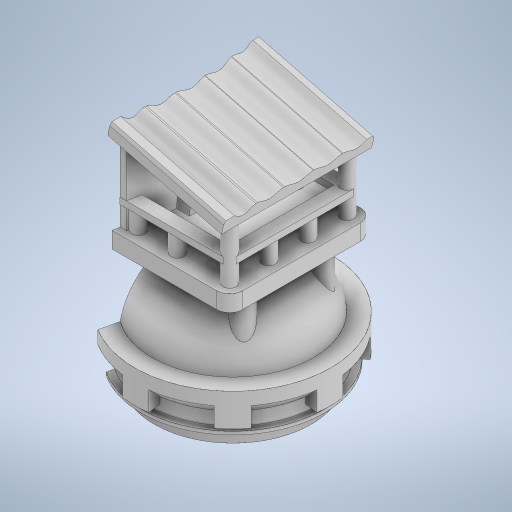
# Autodesk Inventor part: 不知道取啥
Saved by Autodesk Inventor 2024 (Build 280153000, 153)
## iProperties
Created: 2024-05-19
Part Number: 不知道取啥
Material: 一般
Document SubType Name: Modeling
Designer: User
Density: 1 g/cm^3
Appearance: 預設
Author: User
Autodesk Inventor part; units mm, degrees
ref_plane "YZ Plane" through (0, 0, 0) normal (1, 0, 0) x (0, 1, 0)
ref_plane "XZ Plane" through (0, 0, 0) normal (0, 1, 0) x (-1, 0, 0)
ref_plane "XY Plane" through (0, 0, 0) normal (0, 0, 1) x (1, 0, 0)
sketch "草圖1" plane through (0, 0, 0) normal (0, 1, 0) x (-1, 0, 0)
  circle A0 centre (0, 0) radius 15
  dimension "d0" = 30
  constraints: 1 centre point, 1 coincident
  measures "d0" diameter of A0
extrude "擠出1" add sketch "草圖1" along normal blind 2
sketch "草圖2" plane through (0, 0, 0) normal (0, 0, 1) x (1, 0, 0)
  line L0 (0, 0) -> (0, -2)
  line L1 (15, 0) -> (-15, 0) projected
  line L2 (0, -2) -> (13, -2)
  line L3 (13, -2) -> (15, 0)
  dimension "d3" = 2
  dimension "d5" = 13
  constraints: 6 end point, 1 horizontal, 1 vertical
  measures "d3" distance of L0.start L0.end
  measures "d5" distance of L0.end L2.end
sketch "草圖3" plane through (0, 0, 0) normal (0, -1, 0) x (1, 0, 0)
  circle A0 centre (0, 0) radius 15
  circle A1 centre (0, 0) radius 13
  line L0 (0, 0) -> (2, 14.866069)
  line L1 (0, 0) -> (-2, 14.866069)
  line L2 (-2, 14.866069) -> (2, 14.866069)
  line L3 (0, 0) -> (-9.097684, 11.926112)
  line L4 (0, 0) -> (-11.926112, 9.097684)
  line L5 (0, 0) -> (-14.866069, 2)
  line L6 (0, 0) -> (-14.866069, -2)
  line L7 (0, 0) -> (-11.926112, -9.097684)
  line L8 (0, 0) -> (-9.097684, -11.926112)
  line L9 (0, 0) -> (-2, -14.866069)
  line L10 (0, 0) -> (2, -14.866069)
  line L11 (0, 0) -> (9.097684, -11.926112)
  line L12 (0, 0) -> (11.926112, -9.097684)
  line L13 (0, 0) -> (14.866069, -2)
  line L14 (0, 0) -> (14.866069, 2)
  line L15 (0, 0) -> (11.926112, 9.097684)
  line L16 (0, 0) -> (9.097684, 11.926112)
  point P0 (1.733333, -12.883926)
  point P1 (-1.733333, -12.883926)
  point P2 (-7.88466, -10.335963)
  point P3 (-10.335963, -7.88466)
  point P4 (-12.883926, -1.733333)
  point P5 (-12.883926, 1.733333)
  point P6 (10.335963, -7.88466)
  point P7 (7.88466, -10.335963)
  point P8 (12.883926, 1.733333)
  point P9 (12.883926, -1.733333)
  point P10 (7.88466, 10.335963)
  point P11 (10.335963, 7.88466)
  point P12 (-10.335963, 7.88466)
  point P13 (-7.88466, 10.335963)
  point P14 (-1.733333, 12.883926)
  point P15 (1.733333, 12.883926)
  dimension "d4" = 30
  dimension "d6" = 26
  dimension "d7" = 4
  dimension "d8" = 82.3377
  dimension "d9" = 82.3377
  dimension "d12" = 360
  constraints: 34 end point, 4 coincident, 2 centre point, 2 point on circle, 1 horizontal, 39 other
  measures "d4" diameter of A0
  measures "d6" diameter of A1
  measures "d7" distance of L0.end L1.end
  measures "d8" angle of L0 L2
  measures "d9" angle of L1 L2
extrude "擠出2" add sketch "草圖3" along normal blind 3 contours A0 L13 A1 L14 | L15 A1 L16 A0 | A0 L11 A1 L12 | L2 A0 | L0 A1 L1 L2 | A1 L4 A0 L3 | A1 L6 A0 L5 | A1 L8 A0 L7 | A1 L10 A0 L9
revolve "迴轉1" add sketch "草圖2" angle 360 about axis through (0, 0, 0) along (0, -1, 0)
sketch "草圖4" plane through (0, -2, 0) normal (0, -1, 0) x (1, 0, 0)
  circle A0 centre (0, 0) radius 13
  dimension "d17" = 26
  constraints: 1 centre point, 1 coincident
  measures "d17" diameter of A0
extrude "擠出3" add sketch "草圖4" along normal blind 2
sketch "草圖5" plane through (0, -4, 0) normal (0, -1, 0) x (1, 0, 0)
  circle A0 centre (0, 0) radius 14
  dimension "d20" = 28
  constraints: 1 centre point, 1 coincident
  measures "d20" diameter of A0
extrude "擠出4" add sketch "草圖5" along normal blind 0.5
sketch "草圖6" plane through (0, 0, 0) normal (1, 0, 0) x (0, 1, 0)
  line L0 (-4.5, 14) -> (-4.5, -14) projected
  line L1 (-4.5, 0) -> (-4.5, -13)
  line L2 (-4.5, -13) -> (-7, -12)
  line L3 (-7, -12) -> (-7, 0)
  line L4 (-7, 0) -> (-4.5, 0)
  point P0 (0, 0)
  dimension "d23" = 13
  dimension "d24" = 12
  dimension "d25" = 2.5
  constraints: 8 end point, 1 midpoint, 1 parallel, 1 perpendicular, 1 point on line
  measures "d23" distance of L1.start L1.end
  measures "d24" distance of L2.end L3.end
  measures "d25" distance between parallel lines of L0 L3
revolve "迴轉2" add sketch "草圖6" angle 360 about axis through (0, -7, 0) along (0, 1, 0)
ref_plane "工作平面1" through (0, 0, 0) normal (0, 1, 0) x (1, 0, 0)
sketch "草圖7" plane through (0, 0, 0) normal (0, 1, 0) x (1, 0, 0)
  circle A0 centre (0, 0) radius 12.5
  line L0 (-12.5, 0) -> (13, 0)
  arc A1 (12.883926, -1.733333) -> (12.883926, 1.733333) centre (0, 0) ccw
  point P0 (12.5, 0)
  dimension "d28" = 25
  constraints: 2 end point, 1 coincident, 1 horizontal, 1 point on circle, 3 other
revolve "迴轉3" add sketch "草圖7" angle 180 about axis through (-12.5, 0, 0) along (1, 0, 0) picked at (-2.404316, 7.656061) contours L0 A0
sketch "草圖8" plane through (0, 2, 0) normal (0, 1, 0) x (1, 0, 0)
  circle A0 centre (7.515021, -6) radius 1.5
  circle A1 centre (7.515021, 6) radius 1.5
  line L0 (0, 0) -> (8.693271, 0)
  dimension "d30" = 3
  dimension "d31" = 3
  dimension "d32" = 6
  dimension "d33" = 6
  constraints: 2 centre point, 2 end point, 1 horizontal
  measures "d30" diameter of A0
  measures "d31" diameter of A1
  measures "d32" distance from line of L0 A0.centre
  measures "d33" distance from line of L0 A1.centre
extrude "擠出5" add sketch "草圖8" along normal blind 10
sketch "草圖9" plane through (7.515021, 12, 6) normal (0, 1, 0) x (1, 0, 0)
  line L0 (1, -5) -> (-15, -5)
  line L1 (-15, -5) -> (-15, 17)
  line L2 (-15, 17) -> (1, 17)
  line L3 (3, 15) -> (3, -3)
  arc A0 (1, -5) -> (3, -3) centre (1, -3) ccw
  arc A1 (3, 15) -> (1, 17) centre (1, 15) ccw
  circle A2 centre (0, 0) radius 1.5
  circle A3 centre (0, 12) radius 1.5
  line L4 (0, 0) -> (0, 12)
  line L5 (0, 6) -> (-5.052859, 6)
  point P0 (-7.515021, 6)
  point P1 (3, -5)
  dimension "d36" = 22
  dimension "d37" = 18
  dimension "d38" = 2
  dimension "d39" = 11
  dimension "d40" = 3
  constraints: 12 end point, 4 point on circle, 4 tangent, 2 centre point, 2 horizontal, 2 parallel, 2 point on line, 1 equal radius, 1 midpoint, 1 perpendicular, 1 vertical
  measures "d36" distance of L0.end L1.end
  measures "d37" distance of point (3, -5) L0.end
  measures "d38" radius of A0
  measures "d39" distance between parallel lines of L2 L5
  measures "d40" distance between parallel lines of L4 L3
extrude "擠出6" add sketch "草圖9" along normal blind 2.5 contours L0 L1 L2 A1 L3 A0 | A2 | A3
sketch "草圖10" plane through (7.515021, 14.5, 6) normal (0, 1, 0) x (1, 0, 0)
  circle A0 centre (1, -3) radius 1
  circle A1 centre (1, 15) radius 1
  arc A2 (1, -5) -> (3, -3) centre (1, -3) ccw projected
  arc A3 (3, 15) -> (1, 17) centre (1, 15) ccw projected
  circle A4 centre (-7, -3) radius 1
  circle A5 centre (-13, -3) radius 1
  circle A6 centre (1, 3) radius 1
  circle A7 centre (1, 9) radius 1
  circle A8 centre (-7, 15) radius 1
  circle A9 centre (-13, 15) radius 1
  point P0 (-7.515021, 6)
  dimension "d43" = 2
  dimension "d44" = 2
  dimension "d45" = 2
  dimension "d46" = 2
  dimension "d47" = 2
  dimension "d48" = 2
  dimension "d49" = 6
  dimension "d50" = 6
  dimension "d51" = 8
  dimension "d52" = 6
  dimension "d53" = 2
  dimension "d54" = 2
  constraints: 8 centre point, 2 concentric
  measures "d43" diameter of A0
  measures "d44" diameter of A1
  measures "d45" diameter of A4
  measures "d46" diameter of A5
  measures "d47" diameter of A6
  measures "d48" diameter of A7
  measures "d49" distance of A0.centre A6.centre
  measures "d50" distance of A1.centre A7.centre
  measures "d51" distance of A4.centre A0.centre
  measures "d52" distance of A5.centre A4.centre
  measures "d53" diameter of A8
  measures "d54" diameter of A9
extrude "擠出7" add sketch "草圖10" along normal blind 3
sketch "草圖11" plane through (8.515021, 17.5, -9) normal (0, 1, 0) x (1, 0, 0)
  circle A0 centre (0, -18) radius 1
  line L0 (1, -18) -> (1, 0)
  circle A1 centre (0, 0) radius 1
  line L1 (0, 1) -> (-15.99965, 1)
  line L2 (0, 2) -> (-16, 2)
  line L3 (-15.99965, 1) -> (-15.99965, -1)
  line L4 (-1, -12.008919) -> (-1, -1)
  line L5 (-1, -1) -> (-15.99965, -1)
  line L6 (0, -19) -> (-16, -19)
  line L7 (-16, -19) -> (-16, -17)
  line L8 (-16, -17) -> (-1, -17)
  line L9 (-1, -17) -> (-1, -12.008919)
  circle A2 centre (0, 0) radius 1
  circle A3 centre (0, -18) radius 1
  point P0 (-8.515021, -9)
  point P1 (0, 1)
  dimension "d57" = 2
  dimension "d58" = 2
  constraints: 18 end point, 4 perpendicular, 3 point on circle, 3 tangent, 2 parallel, 2 vertical, 1 collinear, 1 point on line, 2 other
  measures "d57" distance of L1.end L3.end
  measures "d58" distance of L6.end L7.end
extrude "擠出8" add sketch "草圖11" along normal blind 1
sketch "草圖12" plane through (8.515021, 18.5, -9) normal (0, 1, 0) x (1, 0, 0)
  circle A0 centre (0, 0) radius 1
  arc A1 (1, -18) -> (0, -19) centre (0, -18) ccw projected
  circle A2 centre (0, -18) radius 1
  point P0 (-8.515021, -9)
  constraints: 2 centre point, 1 coincident
extrude "擠出9" add sketch "草圖12" along normal blind 4.9
ref_plane "工作平面2" through (8.515021, 17.5, 0) normal (0, 0, -1) x (-1, 0, 0)
sketch "草圖13" plane through (8.515021, 17.5, 0) normal (0, 0, -1) x (-1, 0, 0)
  line L0 (-1.734486, 7.276923) -> (-1.240987, 5.338764)
  line L1 (-1.240987, 5.338764) -> (16.202441, 9.78025)
  line L2 (-1.734486, 7.276923) -> (15.708943, 11.718409)
  line L3 (15.708943, 11.718409) -> (16.202441, 9.78025)
  point P0 (8.515021, -17.5)
  dimension "d63" = 2
  dimension "d64" = 18
  constraints: 8 end point, 2 perpendicular
  measures "d63" distance of L0.start L0.end
  measures "d64" distance of L0.end L1.end
extrude "擠出10" add sketch "草圖13" along normal mid plane 23
sketch "草圖14" plane through (9.756008, 22.838764, 11.5) normal (0.9690794, -0.2467492, 0) x (0, 0, -1)
  line L0 (0, 2) -> (0, 0)
  line L1 (23, 2) -> (23, 0)
  line L2 (0, 2) -> (23, 2)
  spline S0 degree 4 poles (0, 1.443308) (0.663407, 4.252166) (2.957851, -1.464209) (3.903051, 3.937048) (7.051409, 0.372177) (8.91973, 3.089502) (11.750041, 0.355073) (13.35708, 3.065261) (16.199219, 0.42801) (18.33258, 3.684152) (21.138996, -0.663348) (22.093895, 3.600431) (23, 1.443308) knots 0 0 0 0 0 0.19575269 0.27873908 0.36526432 0.45419408 0.54523059 0.63496708 0.72263478 0.80844947 1 1 1 1 1
  line L3 (0, 1.443308) -> (0, 2.998728)
  line L4 (0, 2.998728) -> (23, 2.998728)
  line L5 (23, 2.998728) -> (23, 1.443308)
  point P0 (11.5, -24.539863)
  point P1 (1.524949, 2)
  point P2 (3.299043, 1.282053)
  point P3 (4.76079, 2)
  point P4 (6.825254, 1.443425)
  point P5 (9.005657, 2)
  point P6 (11.580757, 1.442973)
  point P7 (13.575268, 2)
  point P8 (16.090682, 1.444916)
  point P9 (18.005703, 2)
  point P10 (20.132117, 1.438398)
  point P11 (21.763454, 2)
  constraints: 9 point on line, 6 end point, 1 collinear, 1 perpendicular, 13 other
extrude "擠出11" cut sketch "草圖14" against normal up to surface (18 mm away) contours L2 S0 L0 | L3 L4 L5 L2 S0 | L2 S0 | L1 S0 L2 | L2 S0 | S0 L2 | L2 S0 | S0 L2 picked at (2.731474, 1.714508) picked at (6.56898, 1.710807) picked at (19.952356, 1.729686) picked at (11.061636, 1.725607) picked at (16.033416, 1.77232)
sketch "草圖15" plane through (7.515021, 14.5, 6) normal (0, 1, 0) x (1, 0, 0)
  arc A0 (-15, -5) -> (-15, 17) centre (-66.845926, 6) ccw
  circle A1 centre (-66.845926, 6) radius 53
  point P0 (-7.515021, 6)
  point P1 (-15, 17)
  point P2 (-15, -5)
  dimension "d69" = 53
  constraints: 2 centre point, 2 point on circle, 1 coincident, 1 concentric
  measures "d69" radius of A0
extrude "擠出12" cut sketch "草圖15" along normal through all both and the other way through all
sketch "草圖16" plane through (7.515021, 14.5, 6) normal (0, 1, 0) x (1, 0, 0)
  arc A0 (-15.159909, -5.728414) -> (-15.159909, 17.728414) centre (-7.515021, 6) ccw
  arc A1 (-14.791214, 15.965291) -> (-15.404301, 18.757714) centre (-66.845926, 6) ccw
  arc A2 (-15, -5) -> (-15, 17) centre (-66.845926, 6) ccw
  arc A3 (-14.791214, -3.965291) -> (-14.791214, 15.965291) centre (-66.845926, 6) ccw
  line L0 (-14.791214, 15.965291) -> (-13.791214, 15.965291)
  line L1 (-14.791214, -3.965291) -> (-13.791817, -4)
  line L2 (-14.797871, -4) -> (-13, -4)
  line L3 (-13, 16) -> (-14.797871, 16)
  arc A4 (-13.791817, -4) -> (-13.791817, 16) centre (-65.839871, 6) ccw
  dimension "d72" = 1
  dimension "d73" = 1
  dimension "d74" = 53
  constraints: 6 point on circle, 4 end point, 2 centre point, 2 point on line, 1 horizontal
  measures "d72" distance of L0.start L0.end
  measures "d73" distance of L1.start L1.end
  measures "d74" radius of A4
extrude "擠出13" add sketch "草圖16" along normal blind 13 contours A1 L3 A4 L1 A2
sketch "草圖17" plane through (7.515021, 14.5, 6) normal (0, 1, 0) x (1, 0, 0)
  arc A0 (-13.464744, -2.114555) -> (-13.464744, 14.114555) centre (-65.839871, 6) ccw
  line L0 (-12.839871, 6) -> (-10.839871, 6)
  line L1 (-12.898867, 8.5) -> (-10.898867, 8.5)
  line L2 (-12.898867, 3.5) -> (-10.898867, 3.5)
  arc A1 (-10.898867, 3.5) -> (-10.898867, 8.5) centre (-63.839871, 6) ccw
  arc A2 (-12.898867, 3.5) -> (-12.898867, 8.5) centre (-65.839871, 6) ccw
  point P0 (-7.515021, 6)
  dimension "d80" = 5
  dimension "d81" = 2.5
  dimension "d85" = 2
  dimension "d86" = 2
  dimension "d87" = 2
  constraints: 9 point on circle, 6 end point, 4 horizontal, 2 centre point
  measures "d80" distance between parallel lines of L1 L2
  measures "d81" distance between parallel lines of L1 L0
  measures "d85" distance of L0.start L0.end
  measures "d86" distance of L2.start L2.end
  measures "d87" distance of L1.start L1.end
extrude "擠出14" add sketch "草圖17" along normal blind 8
draft "面拔模1" angle 5 pull direction (0, 1, 0) fixed plane through (-4.66474, 22.5, -0.277869) normal (0, 1, 0) faces at (-4.050512, 17.166667, -2.5) (-4.717179, 19.833333, 2.5)
